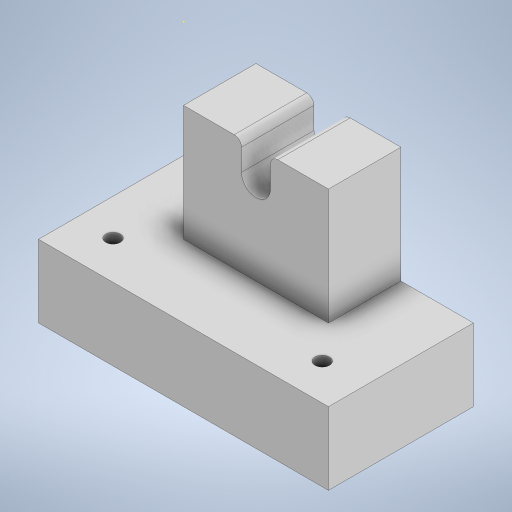
# Autodesk Inventor part: swiatlowod_uchwyt
Saved by Autodesk Inventor 2023 (Build 270158000, 158)
## iProperties
Created: 2022-12-18
Part Number: swiatlowod_uchwyt
Material: Generic
Document SubType Name: Sheet Metal
Designer: KaczorDonald
Density: 1 g/cm^3
Sheet Metal Rule: Default
Appearance: Default
Author: KaczorDonald
Autodesk Inventor part; units mm, degrees
ref_plane "YZ Plane" through (0, 0, 0) normal (1, 0, 0) x (0, 1, 0)
ref_plane "XZ Plane" through (0, 0, 0) normal (0, 1, 0) x (-1, 0, 0)
ref_plane "XY Plane" through (0, 0, 0) normal (0, 0, 1) x (1, 0, 0)
sketch "Sketch1" plane through (0, 0, 0) normal (0, 1, 0) x (-1, 0, 0)
  line L0 (0, 0) -> (-20, 0)
  line L1 (-20, 0) -> (-20, 10)
  line L2 (-20, 10) -> (0, 10)
  line L3 (0, 10) -> (0, 0)
  dimension "d0" = 20
  dimension "d1" = 10
  constraints: 8 end point, 2 parallel, 1 horizontal, 1 perpendicular
  measures "d0" distance of L1.end L2.end
  measures "d1" distance of L0.end L1.end
extrude "Extrusion1" add sketch "Sketch1" along normal blind 5
sketch "Sketch2" plane through (0, 5, 0) normal (0, 1, 0) x (1, 0, 0)
  line L0 (20, 0) -> (0, 0) projected
  line L1 (4.9996, 0) -> (14.9996, 0)
  line L2 (14.9996, 0) -> (14.9996, -5)
  line L3 (14.9996, -5) -> (4.9996, -5)
  line L4 (4.9996, -5) -> (4.9996, 0)
  dimension "d4" = 10
  dimension "d5" = 5
  constraints: 8 end point, 2 parallel, 1 horizontal, 1 perpendicular, 1 point on line
  measures "d4" distance of L2.end L3.end
  measures "d5" distance of L1.end L2.end
extrude "Extrusion2" add sketch "Sketch2" along normal blind 8
sketch "Sketch3" plane through (0, 13, 0) normal (0, 1, 0) x (1, 0, 0)
  point P0 (0, 0)
sketch "Sketch4" plane through (4.9996, 5, 5) normal (0, 0, 1) x (1, 0, 0)
  circle A0 centre (5, 5.9999) radius 1
  point P0 (-4.9996, -5)
  dimension "d8" = 2
  constraints: 1 centre point
  measures "d8" diameter of A0
hole "Hole1" at (9.9996, 10.9999, 5) direction (0, 0, -1) diameter 2 end through all
sketch "Sketch5" plane through (4.9996, 5, 5) normal (0, 0, 1) x (1, 0, 0)
  circle A0 centre (5, 5.9999) radius 1 projected
  line L0 (10, 8) -> (0, 8) projected
  line L1 (4, 5.9999) -> (5.9994, 5.9999)
  line L2 (5.9994, 5.9999) -> (5.9994, 8)
  line L3 (5.9994, 8) -> (4, 8)
  line L4 (4, 8) -> (4, 5.9999)
  point P0 (-4.9996, -5)
  constraints: 8 end point, 2 parallel, 1 horizontal, 1 horizontal alignment, 1 perpendicular, 1 point on line, 1 other
extrude "Extrusion3" cut sketch "Sketch5" against normal blind 5.6375 contours L1 A0 | A0 L4 L0 L2 picked at (5.2495, 6.2209)
sketch "Sketch6" plane through (0, 5, 0) normal (0, 1, 0) x (1, 0, 0)
  circle A0 centre (2.5092, -7.369) radius 0.5
  point P0 (0, 0)
  dimension "d18" = 1
  constraints: 1 centre point
  measures "d18" diameter of A0
hole "Hole2" at (2.5092, 5, 7.369) direction (0, -1, 0) diameter 1 end through all
sketch "Sketch7" plane through (0, 5, 0) normal (0, 1, 0) x (1, 0, 0)
  circle A0 centre (17.0675, -7.4999) radius 0.5
  point P0 (0, 0)
  dimension "d26" = 1
  constraints: 1 centre point
  measures "d26" diameter of A0
hole "Hole3" at (17.0675, 5, 7.4999) direction (0, -1, 0) diameter 1 end through all
fillet "Fillet1" radius 0.5 2 edges at (10.999, 13, 2.5) (8.9996, 13, 2.5)
equation "\"d14\" = Thickness"
equation "\"BendRadius\" = Thickness"
equation "\"BendReliefWidth\" = Thickness"
equation "\"BendReliefDepth\" = 0.5 * Thickness"
equation "\"CornerReliefSize\" = 4 * Thickness"
equation "\"MinimumRemnant\" = 2 * Thickness"
equation "\"TransitionRadius\" = BendRadius"
equation "\"JacobiRadiusSize\" = BendRadius"
equation "\"GapSize\" = Thickness"
equation "\"Thickness\" = 3.048"
body "Solid1"
